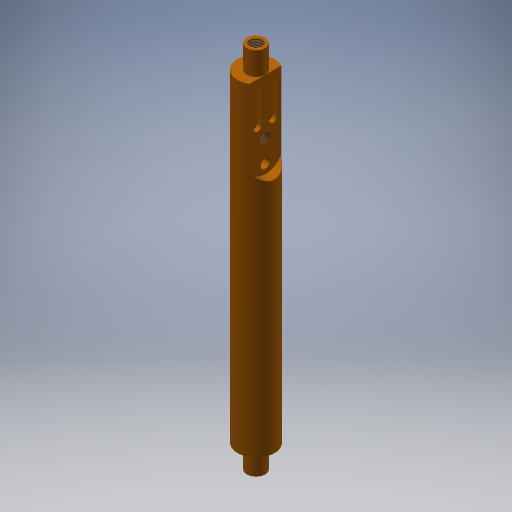
# Autodesk Inventor part: 24_0497_004
Saved by Autodesk Inventor 2024.3 (Build 283343000, 343)
## iProperties
Created: 2024-05-29
Part Number: 24_0497_004
Material: Allgemein
Document SubType Name: Modeling
Designer: Vogel
Density: 1 g/cm^3
Appearance: Orange
Author: Vogel
Autodesk Inventor part; units mm, degrees
ref_plane "XZ Plane" through (0, 0, 0) normal (0, 1, 0) x (-1, 0, 0)
ref_plane "XY Plane" through (0, 0, 0) normal (0, 0, 1) x (1, 0, 0)
sketch "Skizze1" plane through (0, 0, 0) normal (0, 0, 1) x (1, 0, 0)
  line L0 (-8.4, 0) -> (8.4, 0) projected
  line L1 (0, -8.4) -> (0, 8.4) projected
  circle A0 centre (0, 0) radius 6
  dimension "d0" = 12
  constraints: 1 centre point, 1 coincident
  measures "d0" diameter of A0
extrude "Extrusion1" add sketch "Skizze1" along normal blind 120
sketch "Skizze2" plane through (0, 0, 120) normal (0, 0, 1) x (1, 0, 0)
  circle A0 centre (0, 0) radius 6 projected
  circle A1 centre (0, 0) radius 3
  dimension "d3" = 6
  constraints: 1 centre point, 1 coincident
  measures "d3" diameter of A1
extrude "Extrusion2" cut sketch "Skizze2" against normal blind 7.5
sketch "Skizze3" plane through (0, 0, 0) normal (0, 0, -1) x (-1, 0, 0)
  circle A0 centre (0, 0) radius 6 projected
  circle A1 centre (0, 0) radius 3
  circle A2 centre (0, 0) radius 3 projected
  constraints: 2 concentric, 1 centre point, 1 coincident
extrude "Extrusion3" cut sketch "Skizze3" against normal blind 7.5
sketch "Skizze4" plane through (0, 0, 0) normal (0, 0, -1) x (-1, 0, 0)
  circle A0 centre (0, 0) radius 3 projected
  constraints: 1 coincident
hole "Bohrung1" at (0, 0, 0) direction (0, 0, 1) diameter 4.134 depth 14.2 tip angle 118 thread size "M5x0.8" class "6H" standard "ISO Metric profile"
sketch "Skizze5" plane through (0, 0, 120) normal (0, 0, 1) x (1, 0, 0)
  point P0 (0, 0)
  point P1 (0, 0)
  constraints: 1 coincident
hole "Bohrung2" at (0, 0, 120) direction (0, 0, -1) diameter 4.134 depth 14.2 tip angle 118 thread size "M5x0.8" class "6H" standard "ISO Metric profile"
ref_plane "Arbeitsebene1" through (6, 0, 0) normal (1, 0, 0) x (0, 1, 0)
sketch "Skizze7" plane through (6, 0, 0) normal (1, 0, 0) x (0, 1, 0)
  line L0 (-6, 112.5) -> (6, 112.5) projected
  line L1 (-6, 7.5) -> (-6, 112.5) projected
  line L2 (6, 7.5) -> (6, 112.5) projected
  line L3 (-6, 112.5) -> (6, 112.5)
  line L4 (6, 112.5) -> (6, 90.5)
  line L5 (6, 90.5) -> (-6, 90.5)
  line L6 (-6, 90.5) -> (-6, 112.5)
  arc A0 (-6, 90.5) -> (6, 90.5) centre (0, 90.5) ccw
  line L7 (-8.4, 0) -> (8.4, 0) projected
  line L8 (0, -24) -> (0, 144) projected
  point P0 (0, 0)
  dimension "d22" = 22
  constraints: 8 end point, 2 parallel, 2 point on circle, 2 tangent, 1 centre point, 1 horizontal, 1 perpendicular, 1 point on line
  measures "d22" distance between parallel lines of L5 L0
extrude "Extrusion4" cut sketch "Skizze7" against normal blind 3
sketch "Skizze8" plane through (3, 0, 0) normal (1, 0, 0) x (0, 0, -1)
  line L0 (0, -8.4) -> (0, 8.4) projected
  line L1 (24, 0) -> (-144, 0) projected
  line L2 (-109, -2.5) -> (-99, -2.5) construction
  line L3 (-87.5, -5.1962) -> (-112.5, -5.1962) projected
  line L4 (-99, 2.5) -> (-109, 2.5) construction
  line L5 (-109, -2.5) -> (-99, -2.5) construction
  line L6 (-109, -1.25) -> (-99, -1.25)
  line L7 (-99, -3.75) -> (-109, -3.75)
  arc A0 (-109, -1.25) -> (-109, -3.75) centre (-109, -2.5) ccw
  arc A1 (-99, -3.75) -> (-99, -1.25) centre (-99, -2.5) ccw
  line L8 (-109, 2.5) -> (-99, 2.5) construction
  line L9 (-109, 3.75) -> (-99, 3.75)
  line L10 (-99, 1.25) -> (-109, 1.25)
  arc A2 (-109, 3.75) -> (-109, 1.25) centre (-109, 2.5) ccw
  arc A3 (-99, 1.25) -> (-99, 3.75) centre (-99, 2.5) ccw
  line L11 (-112.5, 0) -> (-112.5, 5.1962) projected
  line L12 (-112.5, -5.1962) -> (-112.5, 0) projected
  point P0 (0, 0)
  point P1 (-104, -2.5)
  point P2 (-104, 2.5)
  dimension "d25" = 5
  dimension "d26" = 2.5
  dimension "d27" = 2.5
  dimension "d28" = 3.5
  dimension "d29" = 3.5
  dimension "d30" = 10
  dimension "d31" = 10
  constraints: 20 end point, 8 point on circle, 8 tangent, 4 centre point, 3 parallel, 2 collinear, 2 midpoint, 1 horizontal, 1 other
  measures "d25" distance between parallel lines of L2 L4
  measures "d26" distance between parallel lines of L10 L9
  measures "d27" distance between parallel lines of L7 L6
  measures "d28" distance from line of L11 L9.start
  measures "d29" distance from line of L12 L6.start
  measures "d30" distance of L7.start L7.end
  measures "d31" distance of L9.start L9.end
extrude "Extrusion5" cut sketch "Skizze8" against normal blind 1.3
sketch "Skizze9" plane through (3, 0, 0) normal (1, 0, 0) x (0, 0, -1)
  line L0 (24, 0) -> (-144, 0) projected
  line L1 (0, -8.4) -> (0, 8.4) projected
  line L2 (-112.5, -5.1962) -> (-112.5, 0) projected
  point P0 (0, 0)
  point P1 (-94.5, 0)
  dimension "d34" = 18
  constraints: 1 point on line
  measures "d34" distance from line of point (-94.5, 0) L2
hole "Bohrung3" at (3, 0, 94.5) direction (-1, 0, 0) diameter 3.242 depth 11.8 tip angle 118 thread size "M4x0.7" class "6H" standard "ISO Metric profile"
sketch "Skizze10" plane through (3, 0, 0) normal (1, 0, 0) x (0, 0, -1)
  line L0 (24, 0) -> (-144, 0) projected
  line L1 (0, -8.4) -> (0, 8.4) projected
  circle A0 centre (-94.5, 0) radius 1.621 projected
  point P0 (0, 0)
  point P1 (-87.5, 0)
  dimension "d42" = 7
  constraints: 1 point on line
  measures "d42" distance of point (-87.5, 0) A0.centre
hole "Bohrung4" at (3, 0, 87.5) direction (-1, 0, 0) diameter 3 end through all
equation "\"d27\" = d26"
equation "\"d29\" = d28"
equation "\"d31\" = d30"
